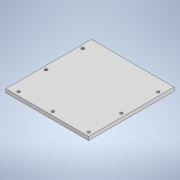
# Autodesk Inventor part: Bottle Base Plate
Saved by Autodesk Inventor 2021 (Build 250183000, 183)
## iProperties
Created: 2020-07-28
Part Number: Bottle Base Plate
Material: Generic
Document SubType Name: Modeling
Designer: jgray
Density: 1 g/cm^3
Appearance: Default
Author: jgray
Autodesk Inventor part; units mm, degrees
ref_plane "YZ Plane" through (0, 0, 0) normal (1, 0, 0) x (0, 1, 0)
ref_plane "XZ Plane" through (0, 0, 0) normal (0, 1, 0) x (-1, 0, 0)
ref_plane "XY Plane" through (0, 0, 0) normal (0, 0, 1) x (1, 0, 0)
sketch "Sketch1" plane through (0, 0, 0) normal (0, 1, 0) x (-1, 0, 0)
  line L0 (-56.25, 58.1) -> (56.25, 58.1)
  line L1 (56.25, 58.1) -> (56.25, -58.1)
  line L2 (56.25, -58.1) -> (-56.25, -58.1)
  line L3 (-56.25, -58.1) -> (-56.25, 58.1)
  line L4 (-56.25, 58.1) -> (56.25, -58.1) construction
  line L5 (56.25, 58.1) -> (-56.25, -58.1) construction
  point P0 (0, 0)
  dimension "d0" = 112.5
  dimension "d1" = 116.2
  constraints: 12 end point, 2 midpoint, 2 parallel, 1 horizontal, 1 perpendicular
  measures "d0" distance of L1.end L2.end
  measures "d1" distance of L0.end L1.end
extrude "Extrusion1" add sketch "Sketch1" along normal blind 5
sketch "Sketch3" plane through (0, 5, 0) normal (0, 1, 0) x (1, 0, 0)
  line L0 (-67.6879, -53.1) -> (61.6788, -53.1) construction
  line L1 (51.25, 64.0604) -> (51.25, -69.5663) construction
  line L2 (-51.25, 74.598) -> (-51.25, -75.8441) construction
  line L3 (-56.25, 58.1) -> (-56.25, -58.1) construction
  line L4 (56.25, -58.1) -> (56.25, 58.1) construction
  line L5 (-56.25, -58.1) -> (56.25, -58.1) construction
  line L6 (-98.6283, 41.4) -> (135.891, 41.4) construction
  line L7 (-92.1264, -8.6) -> (97.1034, -8.6) construction
  line L8 (56.25, 58.1) -> (-56.25, 58.1) construction
  point P0 (0, 0)
  point P1 (51.25, 41.4)
  point P2 (51.25, -8.6)
  point P3 (-51.25, 41.4)
  point P4 (-51.25, -8.6)
  point P5 (-43.95, -53.1)
  point P6 (2.65, -53.1)
  point P7 (51.25, -53.1)
  dimension "d21" = 5
  dimension "d22" = 5
  dimension "d23" = 5
  dimension "d34" = 12.3
  dimension "d35" = 58.9
  dimension "d36" = 107.5
  dimension "d37" = 49.5
  dimension "d38" = 99.5
  constraints: 11 point on line, 10 end point, 3 horizontal, 2 vertical
  measures "d21" distance between parallel lines of L2 L3
  measures "d22" distance between parallel lines of L4 L1
  measures "d23" distance between parallel lines of L5 L0
  measures "d34" distance from line of point (-43.95, -53.1) L3
  measures "d35" distance from line of point (2.65, -53.1) L3
  measures "d36" distance from line of point (51.25, -53.1) L3
  measures "d37" distance between parallel lines of L7 L5
  measures "d38" distance between parallel lines of L6 L5
hole "Hole1" at (51.25, 5, -41.4) at (51.25, 5, 8.6) at (-51.25, 5, -41.4) at (-51.25, 5, 8.6) at (-43.95, 5, 53.1) at (2.65, 5, 53.1) at (51.25, 5, 53.1) direction (0, -1, 0) diameter 3.8 end through all
body "Solid1"
